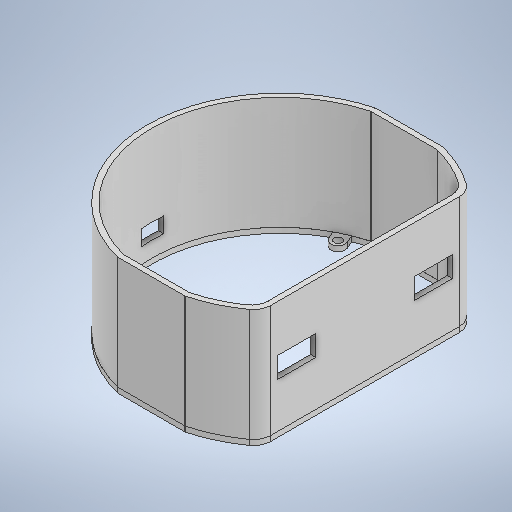
# Autodesk Inventor part: carcasa4.0
Saved by Autodesk Inventor 2025.3 (Build 293356030, 356C)
## iProperties
Created: 2025-08-27
Part Number: carcasa4.0
Material: Generic
Document SubType Name: Modeling
Designer: cdavi
Density: 1 g/cm^3
Appearance: Default
Author: cdavi
Autodesk Inventor part; units mm, degrees
ref_plane "YZ Plane" through (0, 0, 0) normal (1, 0, 0) x (0, 1, 0)
ref_plane "XZ Plane" through (0, 0, 0) normal (0, 1, 0) x (-1, 0, 0)
ref_plane "XY Plane" through (0, 0, 0) normal (0, 0, 1) x (1, 0, 0)
sketch "Sketch1" plane through (0, 0, 0) normal (0, 1, 0) x (-1, 0, 0)
  line L0 (18.8082, 71.5) -> (-18.8082, 71.5)
  line L1 (0, 0) -> (-49, 0) construction
  line L2 (19.2029, 74.5) -> (-19.2029, 74.5)
  line L3 (18.8082, -71.5) -> (-19.0722, -71.5)
  line L4 (19.2029, -74.5) -> (-19.2029, -74.5)
  line L5 (0, 0) -> (0, 74.5) construction
  line L6 (-46, 52.915) -> (-46, -52.915)
  line L7 (-49, 54.4794) -> (-49, -54.4794)
  arc A0 (-41.625, -61.183) -> (-19.0722, -71.5) centre (0, 0) ccw
  arc A1 (-44.8209, -62.6106) -> (-19.7149, -74.4333) centre (0, 0) ccw
  arc A2 (19.7149, -74.4333) -> (19.7149, 74.4333) centre (0, 0) ccw
  arc A3 (-19.7149, 74.4333) -> (-44.8209, 62.6106) centre (0, 0) ccw
  arc A4 (19.3307, -71.4306) -> (19.3307, 71.4306) centre (0, 0) ccw
  arc A5 (-19.3307, 71.4306) -> (-41.625, 61.183) centre (0, 0) ccw
  arc A6 (-19.7149, -74.4333) -> (-19.2029, -74.5) centre (-19.2029, -72.5) ccw
  arc A7 (19.2029, -74.5) -> (19.7149, -74.4333) centre (19.2029, -72.5) ccw
  arc A8 (18.8082, -71.5) -> (19.3307, -71.4306) centre (18.8082, -69.5) ccw
  arc A9 (19.3307, 71.4306) -> (18.8082, 71.5) centre (18.8082, 69.5) ccw
  arc A10 (19.7149, 74.4333) -> (19.2029, 74.5) centre (19.2029, 72.5) ccw
  arc A11 (-18.8082, 71.5) -> (-19.3307, 71.4306) centre (-18.8082, 69.5) ccw
  arc A12 (-19.2029, 74.5) -> (-19.7149, 74.4333) centre (-19.2029, 72.5) ccw
  arc A13 (-41.625, 61.183) -> (-46, 52.915) centre (-36, 52.915) ccw
  arc A14 (-44.8209, 62.6106) -> (-49, 54.4794) centre (-39, 54.4794) ccw
  arc A15 (-49, -54.4794) -> (-44.8209, -62.6106) centre (-39, -54.4794) ccw
  arc A16 (-46, -52.915) -> (-41.625, -61.183) centre (-36, -52.915) ccw
  point P0 (-19.4615, 74.5)
  point P1 (19.0722, -71.5)
  point P2 (19.4615, -74.5)
  point P3 (-19.4615, -74.5)
  point P4 (-49, -59.397)
  point P5 (-46, 57.9655)
  point P6 (-46, -57.9655)
  point P7 (-49, 59.397)
  point P8 (19.4615, 74.5)
  point P9 (19.0722, 71.5)
  point P10 (-19.0722, 71.5)
  dimension "d2" = 71.5
  dimension "d4" = 3
  dimension "d6" = 46
  dimension "d7" = 3
  dimension "d8" = 2
  dimension "d9" = 10
  dimension "d10" = 74
  dimension "d11" = 77
  dimension "d12" = 74
  dimension "d13" = 77
  constraints: 45 point on circle, 22 tangent, 17 centre point, 16 end point, 11 point on line, 9 equal radius, 4 symmetric about line, 3 vertical, 2 coincident, 2 horizontal, 2 midpoint, 1 parallel
  measures "d2" distance between parallel lines of L1 L0
  measures "d4" distance between parallel lines of L0 L2
  measures "d6" distance between parallel lines of L6 L5
  measures "d7" distance between parallel lines of L7 L6
  measures "d8" radius of A6
  measures "d9" radius of A13
  measures "d10" radius of A4
  measures "d11" radius of A2
  measures "d12" radius of A0
  measures "d13" radius of A1
extrude "Extrusion1" add sketch "Sketch1" along normal blind 65
sketch "Sketch2" plane through (49, 0, 54.4794) normal (1, 0, 0) x (0, 0, -1)
  line L0 (54.4794, 0) -> (54.4794, 65) construction
  line L1 (107.3944, 65) -> (1.5643, 65) projected
  line L2 (0, 0) -> (108.9587, 0) projected
  line L3 (-19.954, 0) -> (-19.954, 65) projected
  line L4 (54.4794, 0) -> (54.4794, 65)
  line L5 (54.4794, 0) -> (54.4794, 26)
  line L6 (54.4794, 26) -> (26.0464, 26)
  line L7 (26.0464, 26) -> (26.0464, 38)
  line L8 (26.0464, 38) -> (4.0464, 38)
  line L9 (4.0464, 38) -> (4.0464, 26)
  line L10 (4.0464, 26) -> (26.0464, 26)
  line L11 (82.9124, 26) -> (82.9124, 38)
  line L12 (82.9124, 38) -> (104.9124, 38)
  line L13 (104.9124, 38) -> (104.9124, 26)
  line L14 (104.9124, 26) -> (82.9124, 26)
  dimension "d240" = 26
  dimension "d241" = 28.433
  dimension "d242" = 12
  dimension "d243" = 22
  dimension "d244" = 12
  constraints: 24 end point, 4 symmetric about line, 3 perpendicular, 2 midpoint, 1 point on line, 1 vertical
  measures "d240" distance of L0.start L5.end
  measures "d241" distance of L5.end L6.end
  measures "d242" distance of L6.end L7.end
  measures "d243" distance of L7.end L8.end
  measures "d244" distance of L8.end L9.end
extrude "Extrusion2" cut sketch "Sketch2" against normal blind 13.25
sketch "Sketch3" plane through (49, 0, 54.4794) normal (1, 0, 0) x (0, 0, -1)
  line L0 (3.568, 49.2223) -> (17.7975, 43.9952) construction
  line L1 (2.8909, 47.379) -> (17.1204, 42.1519)
  line L2 (18.4746, 45.8385) -> (4.2452, 51.0656)
  arc A0 (4.2452, 51.0656) -> (2.8909, 47.379) centre (3.568, 49.2223) ccw
  arc A1 (17.1204, 42.1519) -> (18.4746, 45.8385) centre (17.7975, 43.9952) ccw
  arc A2 (44.4296, 11.624) -> (34.6921, 2.9774) centre (43.8866, 2.4292) ccw construction
  arc A3 (44.531, 13.3402) -> (32.9759, 3.0797) centre (43.8866, 2.4292) ccw
  arc A4 (44.3283, 9.9077) -> (36.4083, 2.8751) centre (43.8866, 2.4292) ccw
  arc A5 (44.3283, 9.9077) -> (44.531, 13.3402) centre (44.4296, 11.624) ccw
  arc A6 (32.9759, 3.0797) -> (36.4083, 2.8751) centre (34.6921, 2.9774) ccw
  line L3 (54.4794, 0) -> (54.4794, 65) construction
  line L4 (106.0678, 47.379) -> (91.8383, 42.1519)
  line L5 (90.4841, 45.8385) -> (104.7135, 51.0656)
  arc A7 (106.0678, 47.379) -> (104.7135, 51.0656) centre (105.3907, 49.2223) ccw
  arc A8 (90.4841, 45.8385) -> (91.8383, 42.1519) centre (91.1612, 43.9952) ccw
  point P0 (10.6828, 46.6088)
  constraints: 18 point on circle, 12 end point, 9 centre point, 8 tangent, 6 symmetric about line, 1 midpoint, 1 parallel, 2 other
extrude "Extrusion3" [suppressed]
extrude "Extrusion4" add sketch "Sketch1" along normal blind 3 from surface at 65 separate body contours A9 A4 A8 L3 A0 A16 L6 A13 A5 A11 L0 | A10 A2 A7 L4 A6 A1 A15 L7 A14 A3 A12 L2
sketch "Sketch5" plane through (-19.2029, 68, 74.5) normal (0, 1, 0) x (1, 0, 0)
  circle A0 centre (19.2029, 74.5) radius 8.5
  circle A1 centre (-10.7971, 74.5) radius 2.5
  line L0 (27.3269, 72) -> (36.2029, 72)
  line L1 (36.2029, 72) -> (36.2029, 77)
  line L2 (36.2029, 77) -> (27.3269, 77)
  line L3 (36.2029, 74.5) -> (68.2029, 74.5)
  line L4 (68.2029, 20.0206) -> (68.2029, 128.9794) projected
  line L5 (-10.7971, 74.5) -> (-57.7971, 74.5)
  arc A2 (-0.5121, 148.9333) -> (-0.5121, 0.0667) centre (19.2029, 74.5) ccw projected
  dimension "d26" = 17
  dimension "d27" = 5
  dimension "d31" = 5
  dimension "d32" = 17
  dimension "d47" = 30
  dimension "d204" = 32
  dimension "d205" = 47
  dimension "d206" = 49
  constraints: 10 end point, 3 point on circle, 2 centre point, 2 horizontal alignment, 2 midpoint, 2 perpendicular, 1 coincident, 1 horizontal, 1 point on line
  measures "d26" diameter of A0
  measures "d27" diameter of A1
  measures "d31" distance between parallel lines of L2 L0
  measures "d32" distance from line of A0.centre L1
  measures "d47" distance of A0.centre L5.start
  measures "d204" distance of L3.start L3.end
  measures "d205" distance of L5.start L5.end
  measures "d206" distance from line of L4 point (19.203, 74.5)
extrude "Extrusion5" cut sketch "Sketch5" against normal through all bodies 2
sketch "Sketch6" plane through (0, 0, 0) normal (0, 1, 0) x (-1, 0, 0)
  circle A0 centre (0, 0) radius 69 construction
  arc A1 (-19.3307, 71.4306) -> (-41.625, 61.183) centre (0, 0) ccw projected
  arc A2 (-41.625, 61.183) -> (-46, 52.915) centre (-36, 52.915) ccw projected
  line L0 (-46, -52.915) -> (-46, 52.915) projected
  arc A3 (-46, -52.915) -> (-41.625, -61.183) centre (-36, -52.915) ccw projected
  arc A4 (-41.625, -61.183) -> (-19.0722, -71.5) centre (0, 0) ccw projected
  line L1 (18.8082, -71.5) -> (-19.0722, -71.5) construction
  arc A5 (19.3307, -71.4306) -> (19.3307, 71.4306) centre (0, 0) ccw projected
  line L2 (-18.8082, 71.5) -> (18.8082, 71.5) construction
  line L3 (19.2029, 74.5) -> (-19.2029, 74.5) projected
  arc A6 (-19.7149, 74.4333) -> (-44.8209, 62.6106) centre (0, 0) ccw projected
  arc A7 (-44.8209, 62.6106) -> (-49, 54.4794) centre (-39, 54.4794) ccw projected
  line L4 (-49, 54.4794) -> (-49, -54.4794) projected
  arc A8 (-49, -54.4794) -> (-44.8209, -62.6106) centre (-39, -54.4794) ccw projected
  arc A9 (-44.8209, -62.6106) -> (-19.7149, -74.4333) centre (0, 0) ccw projected
  line L5 (-19.2029, -74.5) -> (19.2029, -74.5) projected
  arc A10 (19.7149, -74.4333) -> (19.7149, 74.4333) centre (0, 0) ccw projected
  arc A11 (-18.5383, 65.4242) -> (-38.25, 56.2222) centre (0, 0) ccw construction
  arc A12 (-38.25, 56.2222) -> (-40, 52.915) centre (-36, 52.915) ccw construction
  line L6 (-40, 52.915) -> (-40, -52.915) construction
  arc A13 (-40, -52.915) -> (-38.25, -56.2222) centre (-36, -52.915) ccw construction
  arc A14 (-38.25, -56.2222) -> (-18.5383, -65.4242) centre (0, 0) ccw construction
  line L7 (-17.9931, -65.5) -> (17.9931, -65.5) construction
  line L8 (-17.9931, 65.5) -> (17.9931, 65.5) construction
  arc A15 (18.5383, -65.4242) -> (18.5383, 65.4242) centre (0, 0) ccw construction
  arc A16 (-8.124, -2.5) -> (-8.124, 2.5) centre (0, 0) ccw projected
  line L9 (0, 0) -> (52.8571, 44.3523) construction
  line L10 (0, 0) -> (77, 0) construction
  line L11 (0, 0) -> (0, -69) construction
  circle A17 centre (29.1607, 62.5352) radius 3 construction
  line L12 (29.1607, 62.5352) -> (0, 0) construction
  circle A18 centre (-29.1607, 62.5352) radius 3 construction
  line L13 (-29.1607, 62.5352) -> (0, 0) construction
  arc A19 (-17.9931, 65.5) -> (-18.5383, 65.4242) centre (-17.9931, 63.5) ccw construction
  arc A20 (-18.5383, -65.4242) -> (-17.9931, -65.5) centre (-17.9931, -63.5) ccw construction
  arc A21 (17.9931, -65.5) -> (18.5383, -65.4242) centre (17.9931, -63.5) ccw construction
  arc A22 (18.5383, 65.4242) -> (17.9931, 65.5) centre (17.9931, 63.5) ccw construction
  arc A23 (-19.7149, -74.4333) -> (-19.2029, -74.5) centre (-19.2029, -72.5) ccw projected
  arc A24 (19.2029, -74.5) -> (19.7149, -74.4333) centre (19.2029, -72.5) ccw projected
  arc A25 (19.7149, 74.4333) -> (19.2029, 74.5) centre (19.2029, 72.5) ccw projected
  arc A26 (-19.2029, 74.5) -> (-19.7149, 74.4333) centre (-19.2029, 72.5) ccw projected
  circle A27 centre (29.1607, -62.5352) radius 3 construction
  circle A28 centre (-29.1607, -62.5352) radius 3 construction
  line L14 (19.3307, 65.1945) -> (19.3307, 71.4306)
  line L15 (-19.3307, 65.1945) -> (-19.3307, 71.4306)
  line L16 (19.3307, 71.4306) -> (-19.3307, 71.4306)
  line L17 (19.3307, -65.1945) -> (19.3307, -71.4306)
  line L18 (-19.3307, -65.1945) -> (-19.3307, -71.4306)
  line L19 (19.3307, -71.4306) -> (-19.3307, -71.4306)
  circle A29 centre (29.1607, 62.5352) radius 4
  circle A30 centre (-29.1607, 62.5352) radius 4
  line L20 (-32.7354, 60.7404) -> (-34.9798, 65.2105)
  circle A31 centre (29.1607, -62.5352) radius 4
  circle A32 centre (-29.1607, -62.5352) radius 4
  line L21 (-32.7354, -60.7404) -> (-34.9798, -65.2105)
  line L22 (32.7354, 60.7404) -> (34.9798, 65.2105)
  line L23 (32.7354, -60.7404) -> (34.9798, -65.2105)
  line L24 (-25.488, 64.1199) -> (-27.4696, 68.7126)
  line L25 (25.488, 64.1199) -> (27.4696, 68.7126)
  line L26 (-25.488, -64.1199) -> (-27.4696, -68.7126)
  line L27 (25.488, -64.1199) -> (27.4696, -68.7126)
  line L28 (-18.8082, 71.5) -> (-49, 71.5)
  line L29 (-49, 71.5) -> (-49, 54.4794)
  line L30 (-28.5788, 71.5) -> (-18.8082, 71.5)
  circle A33 centre (-29.1607, -62.5352) radius 2.25
  circle A34 centre (29.1607, -62.5352) radius 2.25
  circle A35 centre (29.1607, 62.5352) radius 2.25
  circle A36 centre (-29.1607, 62.5352) radius 2.25
  point P0 (-18.2688, -65.5)
  point P1 (-19.3307, 65.1945)
  point P2 (-19.3307, -65.1945)
  point P3 (29.1607, 62.5352)
  point P4 (26.7032, 60.8145)
  point P5 (-46, 24)
  point P6 (-46, 16)
  point P7 (-29.4221, 59.5467)
  point P8 (-19.3307, -71.4306)
  point P9 (-34.9798, -65.2105)
  point P10 (34.9798, -65.2105)
  point P11 (-27.9581, 66.3502)
  point P12 (-27.9581, -66.3502)
  point P13 (27.9581, -66.3502)
  point P14 (27.9581, 66.3502)
  point P15 (-32.8561, 64.0662)
  point P16 (32.8561, -64.0662)
  point P17 (-32.8561, -64.0662)
  point P18 (32.8561, 64.0662)
  point P19 (25.488, -64.1199)
  point P20 (27.4696, -68.7126)
  point P21 (-25.488, -64.1199)
  point P22 (34.0084, -67.0387)
  point P23 (-28.5882, -71.3052)
  point P24 (28.5882, -71.3052)
  point P25 (28.5882, 71.3052)
  point P26 (-28.5882, 71.3052)
  point P27 (34.0084, 67.0387)
  point P28 (-19.3307, -71.4306)
  point P29 (-34.0084, -67.0387)
  point P30 (-34.0084, 67.0387)
  dimension "d33" = 138
  dimension "d229" = 6
  dimension "d34" = 6
  dimension "d35" = 6
  dimension "d36" = 6
  dimension "d37" = 40
  dimension "d38" = 25
  dimension "d42" = 25
  dimension "d44" = 2
  dimension "d62" = 8
  dimension "d64" = 8
  dimension "d171" = 90
  dimension "d172" = 17.0206
  dimension "d227" = 4.5
  dimension "d228" = 4.5
  dimension "d230" = 4.5
  dimension "d231" = 4.5
  constraints: 50 end point, 30 point on circle, 18 centre point, 16 symmetric about line, 12 tangent, 9 coincident, 4 point on line, 3 equal radius, 2 parallel, 1 collinear, 1 horizontal, 1 perpendicular, 1 vertical, 29 other
  measures "d34" radial gap between concentric circles of A1 A11
  measures "d35" distance between parallel lines of L2 L8
  measures "d36" radial gap between concentric circles of A5 A15
  measures "d37" angle of L10 L9
  measures "d38" angle of L11 L12
  measures "d42" angle of L11 L13
  measures "d44" radius of A19
  measures "d62" diameter of A29
  measures "d64" diameter of A30
  measures "d171" angle of L29 L28
  measures "d172" distance of L28.end L4.start
  measures "d227" diameter of A33
  measures "d228" diameter of A34
  measures "d230" diameter of A35
  measures "d231" diameter of A36
extrude "Extrusion6" add sketch "Sketch6" against normal blind 3 separate body contours L24 A30 L20 A1 | A30 | A5 L22 A29 L25 | A29 | A5 L27 A31 L23 | A31 | L21 A32 L26 A4 | A32 | A25 A10 A24 L5 A23 A9 A8 L4 A7 A6 A26 L3
ref_plane "Work Plane2" through (-77, 0, 0) normal (-1, 0, 0) x (0, 0, 1)
sketch "Sketch20" plane through (-77, 0, 0) normal (-1, 0, 0) x (0, 0, 1)
  line L0 (-54.4794, -3) -> (54.4794, -3) projected
  line L1 (0, -3) -> (0, 9)
  line L2 (0, 9) -> (0, 18)
  line L3 (0, 18) -> (6.5, 18)
  line L4 (0, 9) -> (-6.5, 9)
  line L5 (-6.5, 9) -> (6.5, 9)
  line L6 (6.5, 9) -> (6.5, 18)
  line L7 (6.5, 18) -> (-6.5, 18)
  line L8 (-6.5, 18) -> (-6.5, 9)
  point P0 (0, 0)
  dimension "d215" = 12
  dimension "d216" = 9
  dimension "d217" = 6.5
  dimension "d218" = 6.5
  constraints: 16 end point, 3 horizontal, 2 parallel, 2 vertical, 1 midpoint, 1 perpendicular
  measures "d215" distance of L1.start L1.end
  measures "d216" distance of L1.end L2.end
  measures "d217" distance of L2.end L3.end
  measures "d218" distance of L1.end L4.end
extrude "Extrusion16" cut sketch "Sketch20" against normal blind 10.75 bodies 1
body "Solid1"
body "Solid2"
body "Solid3"
